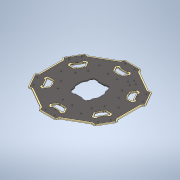
# Autodesk Inventor part: FRAME ATAS
Saved by Autodesk Inventor 2020 (Build 240168000, 168)
## iProperties
Created: 2020-03-27
Part Number: FRAME ATAS
Material: Generic
Document SubType Name: Modeling
Designer: Muhyidin
Density: 1 g/cm^3
Appearance: Carbon Fiber
Author: Muhyidin
Autodesk Inventor part; units mm, degrees
(part 1 of 2)
ref_plane "YZ Plane" through (0, 0, 0) normal (1, 0, 0) x (0, 1, 0)
ref_plane "XZ Plane" through (0, 0, 0) normal (0, 1, 0) x (-1, 0, 0)
ref_plane "XY Plane" through (0, 0, 0) normal (0, 0, 1) x (1, 0, 0)
sketch "Sketch1" plane through (0, 0, 0) normal (0, 1, 0) x (-1, 0, 0)
  circle A0 centre (15.3999, -131.0001) radius 1.6
  circle A1 centre (-15.4001, -131) radius 1.6
  line L0 (-50.3385, -87.1889) -> (-60.4808, -89.9065)
  circle A2 centre (-60.4808, -89.9065) radius 1.5
  line L1 (-50.3385, -87.1889) -> (-40.1963, -84.4713)
  line L2 (-50.3385, -87.1889) -> (-47.6209, -97.3311)
  line L3 (-50.3385, -87.1889) -> (-53.0561, -77.0467)
  circle A3 centre (-53.0561, -77.0467) radius 1.5
  circle A4 centre (-40.1963, -84.4713) radius 1.5
  circle A5 centre (-47.6209, -97.3311) radius 1.5
  line L4 (68.5102, -57.3368) -> (53.5102, -83.3176)
  line L5 (83.9102, -30.6632) -> (98.9102, -4.6824)
  line L6 (-68.5102, 57.3368) -> (-53.5102, 83.3176)
  line L7 (-83.9102, 30.6632) -> (-98.9102, 4.6824)
  line L8 (-83.9102, 30.6632) -> (-53.9102, 30.6632) construction
  circle A6 centre (98.9102, -4.6824) radius 1.6
  circle A7 centre (53.5102, -83.3176) radius 1.6
  circle A8 centre (-98.9102, 4.6824) radius 1.6
  circle A9 centre (-53.5102, 83.3176) radius 1.6
  line L9 (53.5102, -83.3176) -> (68.5102, -83.3176) construction
  circle A10 centre (0, 113) radius 1.6
  line L10 (76.2102, -44) -> (97.8609, -56.5)
  line L11 (76.2102, -44) -> (101.2102, -44) construction
  circle A11 centre (97.8609, -56.5) radius 1.6
  line L12 (-76.2102, -44) -> (-97.8609, -56.5)
  line L13 (-76.2102, -44) -> (-51.2102, -44) construction
  circle A12 centre (-97.8609, -56.5) radius 1.6
  line L14 (25, -145) -> (60, -145) construction
  line L15 (0, -138) -> (25, -138)
  line L16 (0, -138) -> (25, -138) construction
  line L17 (0, -138) -> (-25, -138)
  line L18 (0, -138) -> (25, -138) construction
  line L19 (15.4, -138) -> (22.4, -138) construction
  line L20 (-15.4, -138.0001) -> (-8.4, -138.0001) construction
  line L21 (-25, -138) -> (4.9988, -138) construction
  line L22 (-92.0115, -90.6506) -> (-87.0115, -90.6506) construction
  line L23 (-25, -138) -> (-5.0008, -138) construction
  line L24 (-25, -138) -> (-28.4202, -128.6031)
  line L25 (-25, -138) -> (-15, -138) construction
  line L26 (25, -138) -> (28.4201, -128.6031)
  line L27 (132.0114, -47.3494) -> (125.5835, -39.689)
  line L28 (107.0114, -90.6507) -> (97.1633, -88.9142)
  line L29 (111.8115, -82.3369) -> (115.3115, -76.2747) construction
  line L30 (107.0114, -90.6507) -> (117.011, -73.3308) construction
  line L31 (119.5114, -69) -> (107.0114, -90.6507)
  line L32 (107.0114, -90.6507) -> (122.0108, -64.6709) construction
  line L33 (119.5114, -69) -> (132.0114, -47.3494)
  line L34 (119.5114, -69) -> (132.0114, -47.3494) construction
  line L35 (119.5114, -69) -> (132.0114, -47.3494) construction
  circle A13 centre (121.1493, -52.1634) radius 1.6
  circle A14 centre (105.7492, -78.8369) radius 1.6
  line L36 (107.0114, 90.6505) -> (97.1634, 88.914)
  line L37 (132.0114, 47.3493) -> (125.5835, 39.6888)
  line L38 (127.2115, 55.6631) -> (123.7115, 61.7253) construction
  line L39 (132.0114, 47.3493) -> (122.0118, 64.6691) construction
  line L40 (119.5114, 68.9999) -> (132.0114, 47.3493)
  line L41 (132.0114, 47.3493) -> (117.012, 73.329) construction
  line L42 (119.5114, 68.9999) -> (107.0114, 90.6505)
  line L43 (119.5114, 68.9999) -> (107.0114, 90.6505) construction
  line L44 (119.5114, 68.9999) -> (107.0114, 90.6505) construction
  circle A15 centre (105.7494, 78.8366) radius 1.6
  circle A16 centre (121.1493, 52.163) radius 1.6
  line L45 (-25.0001, 137.9998) -> (-28.4202, 128.6029)
  line L46 (24.9999, 137.9998) -> (28.4202, 128.6029)
  line L47 (15.4, 137.9999) -> (8.4, 137.9999) construction
  line L48 (24.9999, 137.9998) -> (5.0007, 137.9998) construction
  line L49 (-0.0001, 137.9998) -> (24.9999, 137.9998)
  line L50 (24.9999, 137.9998) -> (-4.9989, 137.9998) construction
  line L51 (-0.0001, 137.9998) -> (-25.0001, 137.9998)
  line L52 (-0.0001, 137.9998) -> (-25.0001, 137.9998) construction
  line L53 (-0.0001, 137.9998) -> (-25.0001, 137.9998) construction
  circle A17 centre (-15.3999, 130.9999) radius 1.6
  circle A18 centre (15.4, 130.9999) radius 1.6
  line L54 (-132.0115, 47.3492) -> (-125.5836, 39.6889)
  line L55 (-107.0115, 90.6505) -> (-97.1634, 88.914)
  line L56 (-111.8115, 82.3367) -> (-115.3115, 76.2745) construction
  line L57 (-107.0115, 90.6505) -> (-117.0111, 73.3307) construction
  line L58 (-119.5115, 68.9999) -> (-107.0115, 90.6505)
  line L59 (-107.0115, 90.6505) -> (-122.0109, 64.6707) construction
  line L60 (-119.5115, 68.9999) -> (-132.0115, 47.3492)
  line L61 (-119.5115, 68.9999) -> (-132.0115, 47.3492) construction
  line L62 (-119.5115, 68.9999) -> (-132.0115, 47.3492) construction
  circle A19 centre (-121.1493, 52.1632) radius 1.6
  circle A20 centre (-105.7493, 78.8367) radius 1.6
  line L63 (-107.0114, -90.6507) -> (-97.1634, -88.9142)
  line L64 (-132.0114, -47.3494) -> (-125.5836, -39.689)
  line L65 (-127.2115, -55.6633) -> (-123.7115, -61.7255) construction
  line L66 (-132.0114, -47.3494) -> (-122.0118, -64.6693) construction
  line L67 (-119.5114, -69.0001) -> (-132.0114, -47.3494)
  line L68 (-132.0114, -47.3494) -> (-117.012, -73.3292) construction
  line L69 (-119.5114, -69.0001) -> (-107.0114, -90.6507)
  line L70 (-119.5114, -69.0001) -> (-107.0114, -90.6507) construction
  line L71 (-119.5114, -69.0001) -> (-107.0114, -90.6507) construction
  circle A21 centre (-105.7494, -78.8368) radius 1.6
  circle A22 centre (-121.1493, -52.1632) radius 1.6
  line L72 (-28.4202, -128.6031) -> (-97.1634, -88.9142)
  line L73 (97.1633, -88.9142) -> (28.4201, -128.6031)
  line L74 (125.5835, 39.6888) -> (125.5835, -39.689)
  line L75 (28.4202, 128.6029) -> (97.1634, 88.914)
  line L76 (-97.1634, 88.914) -> (-28.4202, 128.6029)
  line L77 (-125.5836, -39.689) -> (-125.5836, 39.6889)
  line L78 (-15.4, -131) -> (42.1, -131) construction
  circle A23 centre (15.4, -73.5001) radius 1.65
  circle A24 centre (-15.4001, -73.5) radius 1.65
  circle A25 centre (71.3528, -23.4133) radius 1.65
  circle A26 centre (55.9528, -50.0869) radius 1.65
  circle A27 centre (55.9528, 50.0867) radius 1.65
  circle A28 centre (71.3528, 23.413) radius 1.65
  circle A29 centre (-15.4, 73.4999) radius 1.65
  circle A30 centre (15.4, 73.4999) radius 1.65
  circle A31 centre (-71.3529, 23.4131) radius 1.65
  circle A32 centre (-55.9528, 50.0867) radius 1.65
  circle A33 centre (-55.9529, -50.0869) radius 1.65
  circle A34 centre (-71.3529, -23.4132) radius 1.65
  line L79 (36.5897, -0.0001) -> (36.5897, -10.9001)
  line L80 (36.5897, -0.0001) -> (47.4897, -0.0001) construction
  line L81 (36.5897, -10.9001) -> (30.2097, -21.9505)
  line L82 (36.5897, -10.9001) -> (49.3497, -10.9001) construction
  line L83 (30.2097, -21.9505) -> (30.2097, -30.6505)
  line L84 (30.2097, -21.9505) -> (38.9097, -21.9505) construction
  line L85 (30.2097, -30.6505) -> (23.4386, -38.72)
  line L86 (30.2097, -30.6505) -> (40.7437, -30.6505) construction
  line L87 (23.4386, -38.72) -> (12.9386, -38.72)
  line L88 (12.9386, -38.72) -> (11.0102, -36.4219)
  line L89 (0, -88.9499) -> (6, -88.9499)
  line L90 (6, -88.9499) -> (8.5, -88.9499) construction
  line L91 (6, -88.9499) -> (7.9151, -90.5569)
  line L92 (6, -88.9499) -> (8.5, -88.9499) construction
  line L93 (7.9151, -90.5569) -> (14.9151, -90.5569)
  line L94 (14.9151, -90.5569) -> (24.9151, -107.8774)
  line L95 (14.9151, -90.5569) -> (34.9151, -90.5569) construction
  line L96 (24.9151, -107.8774) -> (19.1301, -114.7719)
  line L97 (24.9151, -115.3493) -> (33.9151, -115.3493) construction
  line L98 (19.1301, -114.7719) -> (13.35, -114.7719)
  line L99 (19.1301, -114.7719) -> (24.9101, -114.7719) construction
  line L100 (13.35, -114.7719) -> (11.1, -110.8748)
  line L101 (13.35, -114.7719) -> (17.85, -114.7719) construction
  line L102 (11.1, -110.8748) -> (0, -110.8748)
  line L103 (0, -88.9499) -> (-6, -88.95)
  line L104 (-6, -88.95) -> (-8.5, -88.95) construction
  line L105 (-6, -88.95) -> (-7.9151, -90.557)
  line L106 (-6, -88.95) -> (-8.5, -88.95) construction
  line L107 (-7.9151, -90.557) -> (-14.9151, -90.557)
  line L108 (-14.9151, -90.557) -> (-24.9151, -107.8775)
  line L109 (-14.9151, -90.557) -> (-34.9151, -90.557) construction
  line L110 (-24.9151, -107.8775) -> (-19.13, -114.7719)
  line L111 (-19.13, -114.7719) -> (-13.35, -114.7719)
  line L112 (-19.13, -114.7719) -> (-24.91, -114.7719) construction
  line L113 (-13.35, -114.7719) -> (-11.1, -110.8748)
  line L114 (-13.35, -114.7719) -> (-17.85, -114.7719) construction
  line L115 (-11.1, -110.8748) -> (0, -110.8748)
  line L116 (101.5703, -45.8245) -> (96.0203, -55.4374)
  line L117 (90.4703, -65.0503) -> (96.0203, -55.4374)
  line L118 (92.7203, -68.9474) -> (90.4703, -65.0503)
  line L119 (92.7203, -68.9474) -> (90.4703, -72.8445) construction
  line L120 (70.967, -58.1954) -> (60.967, -75.5159) construction
  line L121 (89.8303, -73.953) -> (86.9403, -78.9587) construction
  line L122 (80.967, -75.5159) -> (89.8303, -73.953)
  line L123 (89.8303, -73.953) -> (92.7203, -68.9474)
  line L124 (70.967, -58.1954) -> (80.967, -75.5159)
  line L125 (77.0328, -44.475) -> (74.0329, -49.6712)
  line L126 (74.0329, -49.6712) -> (72.7829, -51.8362) construction
  line L127 (74.0329, -49.6712) -> (72.7829, -51.8362) construction
  line L128 (74.0329, -49.6712) -> (74.467, -52.1332)
  line L129 (74.467, -52.1332) -> (70.967, -58.1954)
  line L130 (108.9603, -40.8188) -> (111.8503, -35.8132) construction
  line L131 (105.882, -32.3616) -> (108.9603, -40.8188)
  line L132 (85.882, -32.3616) -> (95.882, -15.0411) construction
  line L133 (85.882, -32.3616) -> (105.882, -32.3616)
  line L134 (108.9603, -40.8188) -> (106.0703, -45.8245)
  line L135 (106.0703, -45.8245) -> (108.3203, -41.9274) construction
  line L136 (106.0703, -45.8245) -> (101.5703, -45.8245)
  line L137 (80.0328, -39.2789) -> (81.2828, -37.1138) construction
  line L138 (80.0328, -39.2789) -> (82.382, -38.4238)
  line L139 (80.0328, -39.2789) -> (81.2828, -37.1138) construction
  line L140 (77.0328, -44.475) -> (80.0328, -39.2789)
  line L141 (82.382, -38.4238) -> (85.882, -32.3616)
  line L142 (90.4702, 65.0502) -> (96.0202, 55.4373)
  line L143 (101.5702, 45.8244) -> (96.0202, 55.4373)
  line L144 (106.0702, 45.8244) -> (101.5702, 45.8244)
  line L145 (106.0702, 45.8244) -> (108.3202, 41.9273) construction
  line L146 (85.8821, 32.3615) -> (95.8821, 15.041) construction
  line L147 (108.9603, 40.8188) -> (111.8503, 35.8131) construction
  line L148 (105.8821, 32.3615) -> (108.9603, 40.8188)
  line L149 (108.9603, 40.8188) -> (106.0702, 45.8244)
  line L150 (85.8821, 32.3615) -> (105.8821, 32.3615)
  line L151 (77.0328, 44.4748) -> (80.0328, 39.2788)
  line L152 (80.0328, 39.2788) -> (81.2828, 37.1137) construction
  line L153 (80.0328, 39.2788) -> (81.2828, 37.1137) construction
  line L154 (80.0328, 39.2788) -> (82.3821, 38.4237)
  line L155 (82.3821, 38.4237) -> (85.8821, 32.3615)
  line L156 (89.8302, 73.953) -> (86.9402, 78.9586) construction
  line L157 (80.9669, 75.5157) -> (89.8302, 73.953)
  line L158 (70.9669, 58.1952) -> (60.9669, 75.5157) construction
  line L159 (70.9669, 58.1952) -> (80.9669, 75.5157)
  line L160 (89.8302, 73.953) -> (92.7202, 68.9473)
  line L161 (92.7202, 68.9473) -> (90.4702, 72.8444) construction
  line L162 (92.7202, 68.9473) -> (90.4702, 65.0502)
  line L163 (74.0328, 49.671) -> (72.7828, 51.8361) construction
  line L164 (74.0328, 49.671) -> (74.4669, 52.133)
  line L165 (74.0328, 49.671) -> (72.7828, 51.8361) construction
  line L166 (77.0328, 44.4748) -> (74.0328, 49.671)
  line L167 (74.4669, 52.133) -> (70.9669, 58.1952)
  line L168 (-11.1001, 110.8746) -> (-0.0001, 110.8746)
  line L169 (11.0999, 110.8746) -> (-0.0001, 110.8746)
  line L170 (13.3499, 114.7717) -> (11.0999, 110.8746)
  line L171 (13.3499, 114.7717) -> (17.8499, 114.7717) construction
  line L172 (14.915, 90.5568) -> (34.915, 90.5568) construction
  line L173 (19.13, 114.7717) -> (24.91, 114.7717) construction
  line L174 (24.915, 107.8773) -> (19.13, 114.7717)
  line L175 (19.13, 114.7717) -> (13.3499, 114.7717)
  line L176 (14.915, 90.5568) -> (24.915, 107.8773)
  line L177 (0, 88.9498) -> (5.9999, 88.9498)
  line L178 (5.9999, 88.9498) -> (8.4999, 88.9498) construction
  line L179 (5.9999, 88.9498) -> (8.4999, 88.9498) construction
  line L180 (5.9999, 88.9498) -> (7.915, 90.5568)
  line L181 (7.915, 90.5568) -> (14.915, 90.5568)
  line L182 (-19.1301, 114.7717) -> (-24.9102, 114.7717) construction
  line L183 (-24.9151, 107.8773) -> (-19.1301, 114.7717)
  line L184 (-14.9151, 90.5567) -> (-34.9151, 90.5567) construction
  line L185 (-14.9151, 90.5567) -> (-24.9151, 107.8773)
  line L186 (-19.1301, 114.7717) -> (-13.3501, 114.7717)
  line L187 (-13.3501, 114.7717) -> (-17.8501, 114.7717) construction
  line L188 (-13.3501, 114.7717) -> (-11.1001, 110.8746)
  line L189 (-6, 88.9498) -> (-8.5001, 88.9498) construction
  line L190 (-6, 88.9498) -> (-7.9151, 90.5567)
  line L191 (-6, 88.9498) -> (-8.5, 88.9498) construction
  line L192 (0, 88.9498) -> (-6, 88.9498)
  line L193 (-7.9151, 90.5567) -> (-14.9151, 90.5567)
  line L194 (-101.5703, 45.8243) -> (-96.0203, 55.4372)
  line L195 (-90.4703, 65.0501) -> (-96.0203, 55.4372)
  line L196 (-92.7203, 68.9472) -> (-90.4703, 65.0501)
  line L197 (-92.7203, 68.9472) -> (-90.4703, 72.8443) construction
  line L198 (-70.9671, 58.1952) -> (-60.9671, 75.5157) construction
  line L199 (-89.8303, 73.9529) -> (-86.9403, 78.9585) construction
  line L200 (-80.9671, 75.5157) -> (-89.8303, 73.9529)
  line L201 (-89.8303, 73.9529) -> (-92.7203, 68.9472)
  line L202 (-70.9671, 58.1952) -> (-80.9671, 75.5157)
  line L203 (-77.0329, 44.4748) -> (-74.0329, 49.671)
  line L204 (-74.0329, 49.671) -> (-72.7829, 51.8361) construction
  line L205 (-74.0329, 49.671) -> (-72.7829, 51.8361) construction
  line L206 (-74.0329, 49.671) -> (-74.4671, 52.133)
  line L207 (-74.4671, 52.133) -> (-70.9671, 58.1952)
  line L208 (-108.9604, 40.8187) -> (-111.8504, 35.813) construction
  line L209 (-105.8821, 32.3615) -> (-108.9604, 40.8187)
  line L210 (-85.8821, 32.3615) -> (-95.8821, 15.041) construction
  line L211 (-85.8821, 32.3615) -> (-105.8821, 32.3615)
  line L212 (-108.9604, 40.8187) -> (-106.0703, 45.8243)
  line L213 (-106.0703, 45.8243) -> (-108.3203, 41.9272) construction
  line L214 (-106.0703, 45.8243) -> (-101.5703, 45.8243)
  line L215 (-80.0329, 39.2787) -> (-81.2829, 37.1136) construction
  line L216 (-80.0329, 39.2787) -> (-82.3821, 38.4236)
  line L217 (-80.0329, 39.2787) -> (-81.2829, 37.1136) construction
  line L218 (-77.0329, 44.4748) -> (-80.0329, 39.2787)
  line L219 (-82.3821, 38.4236) -> (-85.8821, 32.3615)
  line L220 (-90.4703, -65.0503) -> (-96.0203, -55.4375)
  line L221 (-101.5703, -45.8246) -> (-96.0203, -55.4375)
  line L222 (-106.0703, -45.8246) -> (-101.5703, -45.8246)
  line L223 (-106.0703, -45.8246) -> (-108.3203, -41.9275) construction
  line L224 (-85.8821, -32.3617) -> (-95.8821, -15.0412) construction
  line L225 (-108.9603, -40.8189) -> (-111.8503, -35.8133) construction
  line L226 (-105.8821, -32.3617) -> (-108.9603, -40.8189)
  line L227 (-108.9603, -40.8189) -> (-106.0703, -45.8246)
  line L228 (-85.8821, -32.3617) -> (-105.8821, -32.3617)
  line L229 (-77.0329, -44.475) -> (-80.0329, -39.2789)
  line L230 (-80.0329, -39.2789) -> (-81.2829, -37.1139) construction
  line L231 (-80.0329, -39.2789) -> (-81.2829, -37.1139) construction
  line L232 (-80.0329, -39.2789) -> (-82.3821, -38.4239)
  line L233 (-82.3821, -38.4239) -> (-85.8821, -32.3617)
  line L234 (-89.8303, -73.9531) -> (-86.9402, -78.9588) construction
  line L235 (-80.967, -75.5159) -> (-89.8303, -73.9531)
  line L236 (-70.967, -58.1954) -> (-60.967, -75.5159) construction
  line L237 (-70.967, -58.1954) -> (-80.967, -75.5159)
  line L238 (-89.8303, -73.9531) -> (-92.7203, -68.9475)
  line L239 (-92.7203, -68.9475) -> (-90.4703, -72.8446) construction
  line L240 (-92.7203, -68.9475) -> (-90.4703, -65.0503)
  line L241 (-74.0329, -49.6712) -> (-72.7829, -51.8363) construction
  line L242 (-74.0329, -49.6712) -> (-74.467, -52.1332)
  line L243 (-74.0329, -49.6712) -> (-72.7829, -51.8362) construction
  line L244 (-77.0329, -44.475) -> (-74.0329, -49.6712)
  line L245 (-74.467, -52.1332) -> (-70.967, -58.1954)
  line L246 (0, -88.9499) -> (0, -36.4219)
  line L247 (0, -91.9499) -> (5.9999, -91.9499)
  line L248 (5.9999, -91.9499) -> (7.532, -93.2355)
  line L249 (5.9999, -91.9499) -> (7.9999, -91.9499) construction
  line L250 (7.532, -93.2355) -> (12.532, -93.2355)
  line L251 (12.532, -93.2355) -> (20.032, -106.2259)
  line L252 (20.032, -106.2259) -> (16.8181, -110.0561)
  line L253 (16.8181, -110.0561) -> (13.8181, -110.0561)
  line L254 (13.8181, -110.0561) -> (12.5681, -107.8911)
  line L255 (12.5681, -107.8911) -> (0, -107.8911)
  line L256 (0, -91.9499) -> (-6, -91.9499)
  line L257 (-6, -91.9499) -> (-7.5321, -93.2355)
  line L258 (-6, -91.9499) -> (-8, -91.9499) construction
  line L259 (-7.5321, -93.2355) -> (-12.5321, -93.2355)
  line L260 (-12.5321, -93.2355) -> (-20.0321, -106.2259)
  line L261 (-20.0321, -106.2259) -> (-16.8181, -110.0561)
  line L262 (-16.8181, -110.0561) -> (-13.8181, -110.0561)
  line L263 (-13.8181, -110.0561) -> (-12.5681, -107.8911)
  line L264 (-12.5681, -107.8911) -> (0, -107.8911)
  line L265 (79.6309, -45.975) -> (76.6309, -51.1711)
  line L266 (76.9782, -53.1407) -> (74.4782, -57.4709)
  line L267 (76.6309, -51.1711) -> (76.9782, -53.1407)
  line L268 (88.4022, -66.9949) -> (87.1522, -64.8299)
  line L269 (87.1522, -64.8299) -> (93.4363, -53.9456)
  line L270 (81.9782, -70.4613) -> (86.9022, -69.593)
  line L271 (86.9022, -69.593) -> (88.4022, -66.9949)
  line L272 (74.4782, -57.4709) -> (81.9782, -70.4613)
  line L273 (82.6309, -40.7789) -> (83.6309, -39.0468) construction
  line L274 (82.6309, -40.7789) -> (84.5103, -40.0949)
  line L275 (79.6309, -45.975) -> (82.6309, -40.7789)
  line L276 (84.5103, -40.0949) -> (87.0103, -35.7647)
  line L277 (87.0103, -35.7647) -> (102.0103, -35.7647)
  line L278 (103.7204, -40.4632) -> (102.2204, -43.0613)
  line L279 (102.2204, -43.0613) -> (99.7204, -43.0613)
  line L280 (102.0103, -35.7647) -> (103.7204, -40.4632)
  line L281 (99.7204, -43.0613) -> (93.4363, -53.9456)
  line L282 (79.6309, 45.9748) -> (82.6309, 40.7787)
  line L283 (84.5103, 40.0947) -> (87.0103, 35.7646)
  line L284 (82.6309, 40.7787) -> (84.5103, 40.0947)
  line L285 (102.2204, 43.0611) -> (99.7204, 43.0611)
  line L286 (99.7204, 43.0611) -> (93.4363, 53.9454)
  line L287 (102.0103, 35.7646) -> (103.7204, 40.463)
  line L288 (103.7204, 40.463) -> (102.2204, 43.0611)
  line L289 (87.0103, 35.7646) -> (102.0103, 35.7646)
  line L290 (76.6309, 51.171) -> (75.6309, 52.903) construction
  line L291 (76.6309, 51.171) -> (76.9782, 53.1406)
  line L292 (79.6309, 45.9748) -> (76.6309, 51.171)
  line L293 (76.9782, 53.1406) -> (74.4782, 57.4707)
  line L294 (74.4782, 57.4707) -> (81.9782, 70.4611)
  line L295 (86.9022, 69.5928) -> (88.4022, 66.9948)
  line L296 (88.4022, 66.9948) -> (87.1522, 64.8297)
  line L297 (81.9782, 70.4611) -> (86.9022, 69.5928)
  line L298 (87.1522, 64.8297) -> (93.4363, 53.9454)
  line L299 (0, 91.9498) -> (5.9999, 91.9498)
  line L300 (7.532, 93.2354) -> (12.532, 93.2354)
  line L301 (5.9999, 91.9498) -> (7.532, 93.2354)
  line L302 (13.8181, 110.056) -> (12.5681, 107.8909)
  line L303 (12.5681, 107.8909) -> (0, 107.8909)
  line L304 (20.032, 106.2257) -> (16.8181, 110.056)
  line L305 (16.8181, 110.056) -> (13.8181, 110.056)
  line L306 (12.532, 93.2354) -> (20.032, 106.2257)
  line L307 (-6, 91.9498) -> (-8, 91.9498) construction
  line L308 (-6, 91.9498) -> (-7.5321, 93.2354)
  line L309 (0, 91.9498) -> (-6, 91.9498)
  line L310 (-7.5321, 93.2354) -> (-12.5321, 93.2354)
  line L311 (-12.5321, 93.2354) -> (-20.0321, 106.2257)
  line L312 (-16.8181, 110.056) -> (-13.8181, 110.056)
  line L313 (-13.8181, 110.056) -> (-12.5681, 107.8909)
  line L314 (-20.0321, 106.2257) -> (-16.8181, 110.056)
  line L315 (-12.5681, 107.8909) -> (0, 107.8909)
  line L316 (-79.6309, 45.9748) -> (-76.631, 51.171)
  line L317 (-76.9783, 53.1406) -> (-74.4783, 57.4707)
  line L318 (-76.631, 51.171) -> (-76.9783, 53.1406)
  line L319 (-88.4023, 66.9948) -> (-87.1523, 64.8297)
  line L320 (-87.1523, 64.8297) -> (-93.4364, 53.9454)
  line L321 (-81.9783, 70.4611) -> (-86.9023, 69.5928)
  line L322 (-86.9023, 69.5928) -> (-88.4023, 66.9948)
  line L323 (-74.4783, 57.4707) -> (-81.9783, 70.4611)
  line L324 (-82.6309, 40.7787) -> (-83.6309, 39.0467) construction
  line L325 (-82.6309, 40.7787) -> (-84.5103, 40.0947)
  line L326 (-79.6309, 45.9748) -> (-82.6309, 40.7787)
  line L327 (-84.5103, 40.0947) -> (-87.0103, 35.7646)
  line L328 (-87.0103, 35.7646) -> (-102.0103, 35.7646)
  line L329 (-103.7204, 40.463) -> (-102.2204, 43.0611)
  line L330 (-102.2204, 43.0611) -> (-99.7204, 43.0611)
  line L331 (-102.0103, 35.7646) -> (-103.7204, 40.463)
  line L332 (-99.7204, 43.0611) -> (-93.4364, 53.9454)
  line L333 (-79.6309, -45.975) -> (-82.6309, -40.7789)
  line L334 (-84.5103, -40.0949) -> (-87.0103, -35.7647)
  line L335 (-82.6309, -40.7789) -> (-84.5103, -40.0949)
  line L336 (-102.2204, -43.0613) -> (-99.7204, -43.0613)
  line L337 (-99.7204, -43.0613) -> (-93.4364, -53.9456)
  line L338 (-102.0103, -35.7647) -> (-103.7204, -40.4632)
  line L339 (-103.7204, -40.4632) -> (-102.2204, -43.0613)
  line L340 (-87.0103, -35.7647) -> (-102.0103, -35.7647)
  line L341 (-76.631, -51.1711) -> (-75.631, -52.9032) construction
  line L342 (-76.631, -51.1711) -> (-76.9783, -53.1407)
  line L343 (-79.6309, -45.975) -> (-76.631, -51.1711)
  line L344 (-76.9783, -53.1407) -> (-74.4783, -57.4709)
  line L345 (-74.4783, -57.4709) -> (-81.9783, -70.4613)
  line L346 (-86.9023, -69.593) -> (-88.4023, -66.9949)
  line L347 (-88.4023, -66.9949) -> (-87.1523, -64.8299)
  line L348 (-81.9783, -70.4613) -> (-86.9023, -69.593)
  line L349 (-87.1523, -64.8299) -> (-93.4364, -53.9456)
  line L350 (0, -138) -> (0, -141)
  line L351 (0, -138) -> (3, -138) construction
  line L352 (-25, -138) -> (-22, -138) construction
  line L353 (-25, -138) -> (-20, -138) construction
  line L354 (0, -141) -> (-27.5173, -141)
  line L355 (0, -141) -> (27.5173, -141) construction
  line L356 (-27.5173, -141) -> (-13.8071, -141) construction
  line L357 (-28.4202, -128.6031) -> (-34.2721, -128.6031)
  line L358 (-28.4202, -128.6031) -> (-22.5683, -128.6031) construction
  line L359 (-107.0114, -90.6507) -> (-104.0114, -90.6507) construction
  line L360 (-27.5173, -141) -> (-30.9375, -131.6031)
  line L361 (-27.5173, -141) -> (-17.5173, -141) construction
  line L362 (0, -141) -> (27.5173, -141)
  line L363 (27.5173, -141) -> (13.8071, -141) construction
  line L364 (27.5173, -141) -> (30.9375, -131.6031)
  line L365 (108.3508, -94.3307) -> (98.5028, -92.5942)
  line L366 (122.1095, -70.5) -> (108.3508, -94.3307)
  line L367 (122.1095, -70.5) -> (135.8681, -46.6693) construction
  line L368 (122.1095, -70.5) -> (135.8681, -46.6693)
  line L369 (135.8681, -46.6693) -> (129.4403, -39.0089)
  line L370 (135.8681, 46.6692) -> (129.4402, 39.0088)
  line L371 (122.1095, 70.4999) -> (135.8681, 46.6692)
  line L372 (122.1095, 70.4999) -> (108.3508, 94.3306) construction
  line L373 (122.1095, 70.4999) -> (108.3508, 94.3306)
  line L374 (108.3508, 94.3306) -> (98.5027, 92.5941)
  line L375 (27.5172, 140.9998) -> (30.9374, 131.6029)
  line L376 (-0.0001, 140.9998) -> (27.5172, 140.9998)
  line L377 (-0.0001, 140.9998) -> (-27.5173, 140.9998) construction
  line L378 (-0.0001, 140.9998) -> (-27.5173, 140.9998)
  line L379 (-27.5173, 140.9998) -> (-30.9376, 131.6029)
  line L380 (-108.3509, 94.3305) -> (-98.5028, 92.5941)
  line L381 (-122.1095, 70.4999) -> (-108.3509, 94.3305)
  line L382 (-122.1095, 70.4999) -> (-135.8682, 46.6692) construction
  line L383 (-122.1095, 70.4999) -> (-135.8682, 46.6692)
  line L384 (-135.8682, 46.6692) -> (-129.4403, 39.0087)
  line L385 (-135.8682, -46.6694) -> (-129.4403, -39.0089)
  line L386 (-122.1095, -70.5001) -> (-135.8682, -46.6694)
  line L387 (-122.1095, -70.5001) -> (-108.3509, -94.3307) construction
  line L388 (-122.1095, -70.5001) -> (-108.3509, -94.3307)
  line L389 (-108.3509, -94.3307) -> (-98.5028, -92.5943)
  line L390 (-30.9375, -131.6031) -> (-98.5028, -92.5943)
  line L391 (98.5028, -92.5942) -> (30.9375, -131.6031)
  line L392 (129.4402, 39.0088) -> (129.4403, -39.0089)
  line L393 (30.9374, 131.6029) -> (98.5027, 92.5941)
  line L394 (-98.5028, 92.5941) -> (-30.9376, 131.6029)
  line L395 (-129.4403, -39.0089) -> (-129.4403, 39.0087)
  line L396 (11.0102, -36.4219) -> (0, -36.4219)
  line L397 (-36.5897, -0.0001) -> (-36.5897, -10.9001)
  line L398 (-36.5897, -10.9001) -> (-30.2097, -21.9505)
  line L399 (-36.5897, -10.9001) -> (-49.3497, -10.9001) construction
  line L400 (-30.2097, -21.9505) -> (-30.2097, -30.6505)
  line L401 (-30.2097, -21.9505) -> (-38.9097, -21.9505) construction
  line L402 (-30.2097, -30.6505) -> (-23.4386, -38.72)
  line L403 (-23.4386, -38.72) -> (-12.9386, -38.72)
  line L404 (-12.9386, -38.72) -> (-11.0102, -36.4219)
  line L405 (-11.0102, -36.4219) -> (0, -36.4219)
  line L406 (36.5897, -0.0001) -> (36.5897, 10.8999)
  line L407 (36.5897, 10.8999) -> (30.2097, 21.9504)
  line L408 (36.5897, 10.8999) -> (49.3497, 10.8999) construction
  line L409 (30.2097, 21.9504) -> (30.2097, 30.6504)
  line L410 (30.2097, 21.9504) -> (38.9097, 21.9504) construction
  line L411 (30.2097, 30.6504) -> (23.4386, 38.7199)
  line L412 (23.4386, 38.7199) -> (12.9386, 38.7199)
  line L413 (12.9386, 38.7199) -> (11.0102, 36.4218)
  line L414 (11.0102, 36.4218) -> (0, 36.4218)
  line L415 (-23.4386, 38.7199) -> (-12.9386, 38.7199)
  line L416 (-30.2097, 30.6504) -> (-23.4386, 38.7199)
  line L417 (-11.0102, 36.4218) -> (0, 36.4218)
  line L418 (-12.9386, 38.7199) -> (-11.0102, 36.4218)
  line L419 (-30.2097, 21.9504) -> (-30.2097, 30.6504)
  line L420 (-30.2097, 21.9504) -> (-38.9097, 21.9504) construction
  line L421 (-36.5897, 10.8999) -> (-30.2097, 21.9504)
  line L422 (-36.5897, 10.8999) -> (-49.3497, 10.8999) construction
  line L423 (-36.5897, -0.0001) -> (-36.5897, 10.8999)
  point P0 (0, -0.0001)
  point P1 (-50.3385, -87.1889)
  point P2 (-50.3385, -87.1889)
  point P3 (-50.3385, -87.1889)
  point P4 (-50.3385, -87.1889)
  point P5 (-50.3385, -87.1889)
  point P6 (28.4201, -128.6031)
  point P7 (-28.4202, 128.6029)
  dimension "d427" = 3.2
  dimension "d428" = 3.2
  dimension "d473" = 10.5
  dimension "d474" = 3
  dimension "d479" = 10.5
  dimension "d480" = 10.5
  dimension "d481" = 10.5
  dimension "d486" = 3
  dimension "d491" = 3
  dimension "d496" = 3
  dimension "d497" = 30
  dimension "d498" = 30
  dimension "d499" = 30
  dimension "d500" = 30
  dimension "d501" = 120
  dimension "d597" = 25
  dimension "d598" = 30
  dimension "d603" = 25
  dimension "d604" = 150
  dimension "d625" = 0
  dimension "d627" = 180
  dimension "d646" = 10
  dimension "d647" = 110
  dimension "d650" = 360
  dimension "d655" = 360
  dimension "d659" = 3.3
  dimension "d664" = 3.3
  dimension "d667" = 360
  dimension "d672" = 10.9
  dimension "d673" = 90
  dimension "d674" = 12.76
  dimension "d675" = 120
  dimension "d676" = 8.7
  dimension "d677" = 90
  dimension "d678" = 10.534
  dimension "d679" = 130
  dimension "d680" = 10.5
  dimension "d681" = 3
  dimension "d684" = 6
  dimension "d687" = 2.5
  dimension "d688" = 40
  dimension "d689" = 7
  dimension "d690" = 20
  dimension "d691" = 60
  dimension "d692" = 9
  dimension "d693" = 129.999
  dimension "d695" = 180
  dimension "d696" = 4.5
  dimension "d697" = 120
  dimension "d701" = 360
  dimension "d705" = 3
  dimension "d706" = 2
  dimension "d707" = 40
  dimension "d708" = 5
  dimension "d709" = 140
  dimension "d710" = 15
  dimension "d711" = 120
  dimension "d712" = 5
  dimension "d713" = 110
  dimension "d714" = 3
  dimension "d715" = 130
  dimension "d716" = 2.5
  dimension "d717" = 120
  dimension "d720" = 360
  constraints: 848 end point, 41 horizontal, 35 centre point, 20 equal length, 10 symmetric about line, 3 parallel, 3 vertical, 2 coincident, 2 perpendicular, 787 other
  measures "d427" diameter of A0
  measures "d428" diameter of A1
  measures "d473" distance of L0.end L0.start
  measures "d474" diameter of A2
  measures "d479" distance of L1.start L1.end
  measures "d480" distance of L1.start L2.end
  measures "d481" distance of L1.start L3.end
  measures "d486" diameter of A3
  measures "d491" diameter of A4
  measures "d496" diameter of A5
  measures "d497" distance of L4.start L4.end
  measures "d498" distance of L5.start L5.end
  measures "d499" distance of L6.start L6.end
  measures "d500" distance of L7.start L7.end
  measures "d501" angle of L7 L8
  measures "d597" distance of L10.start L10.end
  measures "d598" angle of L10 L11
  measures "d603" distance of L12.start L12.end
  measures "d604" angle of L12 L13
  measures "d625" distance between parallel lines of L15 L16
  measures "d627" angle of L17 L18
  measures "d646" distance of L17.end L24.end
  measures "d647" angle of L25 L24
  measures "d659" diameter of A23
  measures "d664" diameter of A24
  measures "d672" distance of L79.start L79.end
  measures "d673" angle of L79 L80
  measures "d674" distance of L79.end L81.end
  measures "d675" angle of L81 L82
  measures "d676" distance of L81.end L83.end
  measures "d677" angle of L83 L84
  measures "d678" distance of L83.end L85.end
  measures "d679" angle of L85 L86
  measures "d680" distance of L85.end L87.end
  measures "d681" distance of L87.end L88.end
  measures "d684" distance of L89.start L89.end
  measures "d687" distance of L89.end L91.end
  measures "d688" angle of L91 L92
  measures "d689" distance of L91.end L93.end
  measures "d690" distance of L93.end L94.end
  measures "d691" angle of L94 L95
  measures "d692" distance of L94.end L96.end
  measures "d693" angle of L96 L97
  measures "d695" angle of L98 L99
  measures "d696" distance of L98.end L100.end
  measures "d697" angle of L101 L100
  measures "d705" distance of L89.start L247.start
  measures "d706" distance of L247.end L248.end
  measures "d707" angle of L248 L249
  measures "d708" distance of L248.end L250.end
  measures "d709" angle of L250 L248
  measures "d710" distance of L250.end L251.end
  measures "d711" angle of L250 L251
  measures "d712" distance of L251.end L252.end
  measures "d713" angle of L251 L252
  measures "d714" distance of L252.end L253.end
  measures "d715" angle of L252 L253
  measures "d716" distance of L253.end L254.end
  measures "d717" angle of L253 L254
extrude "Extrusion11" add sketch "Sketch1" along normal blind 3 contours L17 L24 L72 L63 L69 L67 L64 L77 L54 L60 L58 L55 L76 L45 L51 L49 L46 L75 L36 L42 L40 L37 L74 L27 L33 L31 L28 L73 L26 L15
sketch "Sketch3" plane through (0, 3, 0) normal (0, 1, 0) x (1, 0, 0)
  circle A0 centre (15.3999, -131.0001) radius 1.6
  circle A1 centre (-15.4001, -131) radius 1.6
  circle A2 centre (-60.4808, -89.9065) radius 1.5
  line L0 (-50.3385, -87.1889) -> (-60.4808, -89.9065)
  line L1 (-50.3385, -87.1889) -> (-40.1963, -84.4713)
  line L2 (-50.3385, -87.1889) -> (-47.6209, -97.3311)
  line L3 (-50.3385, -87.1889) -> (-53.0561, -77.0467)
  circle A3 centre (-53.0561, -77.0467) radius 1.5
  circle A4 centre (-40.1963, -84.4713) radius 1.5
  circle A5 centre (-47.6209, -97.3311) radius 1.5
  line L4 (68.5102, -57.3368) -> (53.5102, -83.3176)
  line L5 (83.9102, -30.6632) -> (98.9102, -4.6824)
  line L6 (-68.5102, 57.3368) -> (-53.5102, 83.3176)
  line L7 (-83.9102, 30.6632) -> (-98.9102, 4.6824)
  line L8 (-83.9102, 30.6632) -> (-53.9102, 30.6632) construction
  circle A6 centre (98.9102, -4.6824) radius 1.6
  circle A7 centre (53.5102, -83.3176) radius 1.6
  circle A8 centre (-98.9102, 4.6824) radius 1.6
  circle A9 centre (-53.5102, 83.3176) radius 1.6
  line L9 (53.5102, -83.3176) -> (68.5102, -83.3176) construction
  circle A10 centre (0, 113) radius 1.6
  line L10 (76.2102, -44) -> (97.8609, -56.5)
  line L11 (76.2102, -44) -> (101.2102, -44) construction
  circle A11 centre (97.8609, -56.5) radius 1.6
  line L12 (-76.2102, -44) -> (-97.8609, -56.5)
  line L13 (-76.2102, -44) -> (-51.2102, -44) construction
  circle A12 centre (-97.8609, -56.5) radius 1.6
  line L14 (25, -145) -> (60, -145) construction
  line L15 (0, -138) -> (25, -138)
  line L16 (0, -138) -> (25, -138) construction
  line L17 (0, -138) -> (-25, -138)
  line L18 (0, -138) -> (25, -138) construction
  line L19 (15.4, -138) -> (22.4, -138) construction
  line L20 (-15.4, -138.0001) -> (-8.4, -138.0001) construction
  line L21 (-25, -138) -> (4.9988, -138) construction
  line L22 (-92.0115, -90.6506) -> (-87.0115, -90.6506) construction
  line L23 (-25, -138) -> (-5.0008, -138) construction
  line L24 (-25, -138) -> (-28.4202, -128.6031)
  line L25 (-25, -138) -> (-15, -138) construction
  line L26 (25, -138) -> (28.4201, -128.6031)
  line L27 (132.0114, -47.3494) -> (125.5835, -39.689)
  line L28 (107.0114, -90.6507) -> (97.1633, -88.9142)
  line L29 (111.8115, -82.3369) -> (115.3115, -76.2747) construction
  line L30 (107.0114, -90.6507) -> (117.011, -73.3308) construction
  line L31 (119.5114, -69) -> (107.0114, -90.6507)
  line L32 (107.0114, -90.6507) -> (122.0108, -64.6709) construction
  line L33 (119.5114, -69) -> (132.0114, -47.3494)
  line L34 (119.5114, -69) -> (132.0114, -47.3494) construction
  line L35 (119.5114, -69) -> (132.0114, -47.3494) construction
  circle A13 centre (121.1493, -52.1634) radius 1.6
  circle A14 centre (105.7492, -78.8369) radius 1.6
  line L36 (107.0114, 90.6505) -> (97.1634, 88.914)
  line L37 (132.0114, 47.3493) -> (125.5835, 39.6888)
  line L38 (127.2115, 55.6631) -> (123.7115, 61.7253) construction
  line L39 (132.0114, 47.3493) -> (122.0118, 64.6691) construction
  line L40 (119.5114, 68.9999) -> (132.0114, 47.3493)
  line L41 (132.0114, 47.3493) -> (117.012, 73.329) construction
  line L42 (119.5114, 68.9999) -> (107.0114, 90.6505)
  line L43 (119.5114, 68.9999) -> (107.0114, 90.6505) construction
  line L44 (119.5114, 68.9999) -> (107.0114, 90.6505) construction
  circle A15 centre (105.7494, 78.8366) radius 1.6
  circle A16 centre (121.1493, 52.163) radius 1.6
  line L45 (-25.0001, 137.9998) -> (-28.4202, 128.6029)
  line L46 (24.9999, 137.9998) -> (28.4202, 128.6029)
  line L47 (15.4, 137.9999) -> (8.4, 137.9999) construction
  line L48 (24.9999, 137.9998) -> (5.0007, 137.9998) construction
  line L49 (-0.0001, 137.9998) -> (24.9999, 137.9998)
  line L50 (24.9999, 137.9998) -> (-4.9989, 137.9998) construction
  line L51 (-0.0001, 137.9998) -> (-25.0001, 137.9998)
  line L52 (-0.0001, 137.9998) -> (-25.0001, 137.9998) construction
  line L53 (-0.0001, 137.9998) -> (-25.0001, 137.9998) construction
  circle A17 centre (-15.3999, 130.9999) radius 1.6
  circle A18 centre (15.4, 130.9999) radius 1.6
  line L54 (-132.0115, 47.3492) -> (-125.5836, 39.6889)
  line L55 (-107.0115, 90.6505) -> (-97.1634, 88.914)
  line L56 (-111.8115, 82.3367) -> (-115.3115, 76.2745) construction
  line L57 (-107.0115, 90.6505) -> (-117.0111, 73.3307) construction
  line L58 (-119.5115, 68.9999) -> (-107.0115, 90.6505)
  line L59 (-107.0115, 90.6505) -> (-122.0109, 64.6707) construction
  line L60 (-119.5115, 68.9999) -> (-132.0115, 47.3492)
  line L61 (-119.5115, 68.9999) -> (-132.0115, 47.3492) construction
  line L62 (-119.5115, 68.9999) -> (-132.0115, 47.3492) construction
  circle A19 centre (-121.1493, 52.1632) radius 1.6
  circle A20 centre (-105.7493, 78.8367) radius 1.6
  line L63 (-107.0114, -90.6507) -> (-97.1634, -88.9142)
  line L64 (-132.0114, -47.3494) -> (-125.5836, -39.689)
  line L65 (-127.2115, -55.6633) -> (-123.7115, -61.7255) construction
  line L66 (-132.0114, -47.3494) -> (-122.0118, -64.6693) construction
  line L67 (-119.5114, -69.0001) -> (-132.0114, -47.3494)
  line L68 (-132.0114, -47.3494) -> (-117.012, -73.3292) construction
  line L69 (-119.5114, -69.0001) -> (-107.0114, -90.6507)
  line L70 (-119.5114, -69.0001) -> (-107.0114, -90.6507) construction
  line L71 (-119.5114, -69.0001) -> (-107.0114, -90.6507) construction
  circle A21 centre (-105.7494, -78.8368) radius 1.6
  circle A22 centre (-121.1493, -52.1632) radius 1.6
  line L72 (-28.4202, -128.6031) -> (-97.1634, -88.9142)
  line L73 (97.1633, -88.9142) -> (28.4201, -128.6031)
  line L74 (125.5835, 39.6888) -> (125.5835, -39.689)
  line L75 (28.4202, 128.6029) -> (97.1634, 88.914)
  line L76 (-97.1634, 88.914) -> (-28.4202, 128.6029)
  line L77 (-125.5836, -39.689) -> (-125.5836, 39.6889)
  line L78 (-15.4, -131) -> (42.1, -131) construction
  circle A23 centre (15.4, -73.5001) radius 1.65
  circle A24 centre (-15.4001, -73.5) radius 1.65
  circle A25 centre (71.3528, -23.4133) radius 1.65
  circle A26 centre (55.9528, -50.0869) radius 1.65
  circle A27 centre (55.9528, 50.0867) radius 1.65
  circle A28 centre (71.3528, 23.413) radius 1.65
  circle A29 centre (-15.4, 73.4999) radius 1.65
  circle A30 centre (15.4, 73.4999) radius 1.65
  circle A31 centre (-71.3529, 23.4131) radius 1.65
  circle A32 centre (-55.9528, 50.0867) radius 1.65
  circle A33 centre (-55.9529, -50.0869) radius 1.65
  circle A34 centre (-71.3529, -23.4132) radius 1.65
  line L79 (30, -0.0001) -> (30, -10.9001)
  line L80 (30, -0.0001) -> (40.9, -0.0001) construction
  line L81 (-30, -0.0001) -> (-30, -10.9001)
  line L82 (30, -10.9001) -> (23.62, -21.9505)
  line L83 (30, -10.9001) -> (42.76, -10.9001) construction
  line L84 (23.62, -21.9505) -> (23.62, -30.6505)
  line L85 (23.62, -21.9505) -> (32.32, -21.9505) construction
  line L86 (23.62, -30.6505) -> (16.8489, -38.72)
  line L87 (23.62, -30.6505) -> (34.154, -30.6505) construction
  line L88 (16.8489, -38.72) -> (6.3489, -38.72)
  line L89 (6.3489, -38.72) -> (4.4205, -36.4219)
  line L90 (4.4205, -36.4219) -> (0, -36.4219)
  line L91 (-4.4205, -36.4219) -> (0, -36.4219)
  line L92 (-6.3489, -38.7201) -> (-4.4205, -36.4219)
  line L93 (-16.8489, -38.7201) -> (-6.3489, -38.7201)
  line L94 (-23.62, -30.6506) -> (-16.8489, -38.7201)
  line L95 (-23.62, -21.9506) -> (-23.62, -30.6506)
  line L96 (-30, -10.9001) -> (-23.62, -21.9506)
  line L97 (-30, -0.0001) -> (-30, -10.9001)
  line L98 (30, -0.0001) -> (30, 10.8999)
  line L99 (30, 10.8999) -> (23.62, 21.9504)
  line L100 (23.62, 21.9504) -> (23.62, 30.6504)
  line L101 (23.62, 30.6504) -> (16.8488, 38.7199)
  line L102 (16.8488, 38.7199) -> (6.3488, 38.7199)
  line L103 (6.3488, 38.7199) -> (4.4205, 36.4218)
  line L104 (4.4205, 36.4218) -> (0, 36.4218)
  line L105 (-16.8489, 38.7199) -> (-6.3489, 38.7199)
  line L106 (-6.3489, 38.7199) -> (-4.4205, 36.4218)
  line L107 (-4.4205, 36.4218) -> (0, 36.4218)
  line L108 (-23.62, 30.6504) -> (-16.8489, 38.7199)
  line L109 (-23.62, 21.9504) -> (-23.62, 30.6504)
  line L110 (-30, 10.8999) -> (-23.62, 21.9504)
  line L111 (-30, -0.0001) -> (-30, 10.8999)
  line L112 (-30, -0.0001) -> (-30, 10.8999)
  line L113 (0, -88.9499) -> (6, -88.9499)
  line L114 (6, -88.9499) -> (8.5, -88.9499) construction
  line L115 (6, -88.9499) -> (7.9151, -90.5569)
  line L116 (6, -88.9499) -> (8.5, -88.9499) construction
  line L117 (7.9151, -90.5569) -> (14.9151, -90.5569)
  line L118 (14.9151, -90.5569) -> (24.9151, -107.8774)
  line L119 (14.9151, -90.5569) -> (34.9151, -90.5569) construction
  line L120 (24.9151, -107.8774) -> (19.1301, -114.7719)
  line L121 (24.9151, -115.3493) -> (33.9151, -115.3493) construction
  line L122 (19.1301, -114.7719) -> (13.35, -114.7719)
  line L123 (19.1301, -114.7719) -> (24.9101, -114.7719) construction
  line L124 (13.35, -114.7719) -> (11.1, -110.8748)
  line L125 (13.35, -114.7719) -> (17.85, -114.7719) construction
  line L126 (11.1, -110.8748) -> (0, -110.8748)
  line L127 (-11.1, -110.8748) -> (0, -110.8748)
  line L128 (-13.35, -114.7719) -> (-17.85, -114.7719) construction
  line L129 (-19.13, -114.7719) -> (-13.35, -114.7719)
  line L130 (0, -88.9499) -> (-6, -88.95)
  line L131 (-6, -88.95) -> (-7.9151, -90.557)
  line L132 (-6, -88.95) -> (-8.5, -88.95) construction
  line L133 (-6, -88.95) -> (-8.5, -88.95) construction
  line L134 (-7.9151, -90.557) -> (-14.9151, -90.557)
  line L135 (-19.13, -114.7719) -> (-24.91, -114.7719) construction
  line L136 (-24.9151, -107.8775) -> (-19.13, -114.7719)
  line L137 (-14.9151, -90.557) -> (-24.9151, -107.8775)
  line L138 (-14.9151, -90.557) -> (-34.9151, -90.557) construction
  line L139 (-13.35, -114.7719) -> (-11.1, -110.8748)
  line L140 (101.5703, -45.8245) -> (96.0203, -55.4374)
  line L141 (90.4703, -65.0503) -> (96.0203, -55.4374)
  line L142 (92.7203, -68.9474) -> (90.4703, -65.0503)
  line L143 (92.7203, -68.9474) -> (90.4703, -72.8445) construction
  line L144 (70.967, -58.1954) -> (60.967, -75.5159) construction
  line L145 (89.8303, -73.953) -> (86.9403, -78.9587) construction
  line L146 (80.967, -75.5159) -> (89.8303, -73.953)
  line L147 (89.8303, -73.953) -> (92.7203, -68.9474)
  line L148 (70.967, -58.1954) -> (80.967, -75.5159)
  line L149 (77.0328, -44.475) -> (74.0329, -49.6712)
  line L150 (74.0329, -49.6712) -> (72.7829, -51.8362) construction
  line L151 (74.0329, -49.6712) -> (72.7829, -51.8362) construction
  line L152 (74.0329, -49.6712) -> (74.467, -52.1332)
  line L153 (74.467, -52.1332) -> (70.967, -58.1954)
  line L154 (108.9603, -40.8188) -> (111.8503, -35.8132) construction
  line L155 (105.882, -32.3616) -> (108.9603, -40.8188)
  line L156 (85.882, -32.3616) -> (95.882, -15.0411) construction
  line L157 (85.882, -32.3616) -> (105.882, -32.3616)
  line L158 (108.9603, -40.8188) -> (106.0703, -45.8245)
  line L159 (106.0703, -45.8245) -> (108.3203, -41.9274) construction
  line L160 (106.0703, -45.8245) -> (101.5703, -45.8245)
  line L161 (80.0328, -39.2789) -> (81.2828, -37.1138) construction
  line L162 (80.0328, -39.2789) -> (82.382, -38.4238)
  line L163 (80.0328, -39.2789) -> (81.2828, -37.1138) construction
  line L164 (77.0328, -44.475) -> (80.0328, -39.2789)
  line L165 (82.382, -38.4238) -> (85.882, -32.3616)
  line L166 (90.4702, 65.0502) -> (96.0202, 55.4373)
  line L167 (101.5702, 45.8244) -> (96.0202, 55.4373)
  line L168 (106.0702, 45.8244) -> (101.5702, 45.8244)
  line L169 (106.0702, 45.8244) -> (108.3202, 41.9273) construction
  line L170 (85.8821, 32.3615) -> (95.8821, 15.041) construction
  line L171 (108.9603, 40.8188) -> (111.8503, 35.8131) construction
  line L172 (105.8821, 32.3615) -> (108.9603, 40.8188)
  line L173 (108.9603, 40.8188) -> (106.0702, 45.8244)
  line L174 (85.8821, 32.3615) -> (105.8821, 32.3615)
  line L175 (77.0328, 44.4748) -> (80.0328, 39.2788)
  line L176 (80.0328, 39.2788) -> (81.2828, 37.1137) construction
  line L177 (80.0328, 39.2788) -> (81.2828, 37.1137) construction
  line L178 (80.0328, 39.2788) -> (82.3821, 38.4237)
  line L179 (82.3821, 38.4237) -> (85.8821, 32.3615)
  line L180 (89.8302, 73.953) -> (86.9402, 78.9586) construction
  line L181 (80.9669, 75.5157) -> (89.8302, 73.953)
  line L182 (70.9669, 58.1952) -> (60.9669, 75.5157) construction
  line L183 (70.9669, 58.1952) -> (80.9669, 75.5157)
  line L184 (89.8302, 73.953) -> (92.7202, 68.9473)
  line L185 (92.7202, 68.9473) -> (90.4702, 72.8444) construction
  line L186 (92.7202, 68.9473) -> (90.4702, 65.0502)
  line L187 (74.0328, 49.671) -> (72.7828, 51.8361) construction
  line L188 (74.0328, 49.671) -> (74.4669, 52.133)
  line L189 (74.0328, 49.671) -> (72.7828, 51.8361) construction
  line L190 (77.0328, 44.4748) -> (74.0328, 49.671)
  line L191 (74.4669, 52.133) -> (70.9669, 58.1952)
  line L192 (-11.1001, 110.8746) -> (-0.0001, 110.8746)
  line L193 (11.0999, 110.8746) -> (-0.0001, 110.8746)
  line L194 (13.3499, 114.7717) -> (11.0999, 110.8746)
  line L195 (13.3499, 114.7717) -> (17.8499, 114.7717) construction
  line L196 (14.915, 90.5568) -> (34.915, 90.5568) construction
  line L197 (19.13, 114.7717) -> (24.91, 114.7717) construction
  line L198 (24.915, 107.8773) -> (19.13, 114.7717)
  line L199 (19.13, 114.7717) -> (13.3499, 114.7717)
  line L200 (14.915, 90.5568) -> (24.915, 107.8773)
  line L201 (0, 88.9498) -> (5.9999, 88.9498)
  line L202 (5.9999, 88.9498) -> (8.4999, 88.9498) construction
  line L203 (5.9999, 88.9498) -> (8.4999, 88.9498) construction
  line L204 (5.9999, 88.9498) -> (7.915, 90.5568)
  line L205 (7.915, 90.5568) -> (14.915, 90.5568)
  line L206 (-19.1301, 114.7717) -> (-24.9102, 114.7717) construction
  line L207 (-24.9151, 107.8773) -> (-19.1301, 114.7717)
  line L208 (-14.9151, 90.5567) -> (-34.9151, 90.5567) construction
  line L209 (-14.9151, 90.5567) -> (-24.9151, 107.8773)
  line L210 (-19.1301, 114.7717) -> (-13.3501, 114.7717)
  line L211 (-13.3501, 114.7717) -> (-17.8501, 114.7717) construction
  line L212 (-13.3501, 114.7717) -> (-11.1001, 110.8746)
  line L213 (-6, 88.9498) -> (-8.5001, 88.9498) construction
  line L214 (-6, 88.9498) -> (-7.9151, 90.5567)
  line L215 (-6, 88.9498) -> (-8.5, 88.9498) construction
  line L216 (0, 88.9498) -> (-6, 88.9498)
  line L217 (-7.9151, 90.5567) -> (-14.9151, 90.5567)
  line L218 (-101.5703, 45.8243) -> (-96.0203, 55.4372)
  line L219 (-90.4703, 65.0501) -> (-96.0203, 55.4372)
  line L220 (-92.7203, 68.9472) -> (-90.4703, 65.0501)
  line L221 (-92.7203, 68.9472) -> (-90.4703, 72.8443) construction
  line L222 (-70.9671, 58.1952) -> (-60.9671, 75.5157) construction
  line L223 (-89.8303, 73.9529) -> (-86.9403, 78.9585) construction
  line L224 (-80.9671, 75.5157) -> (-89.8303, 73.9529)
  line L225 (-89.8303, 73.9529) -> (-92.7203, 68.9472)
  line L226 (-70.9671, 58.1952) -> (-80.9671, 75.5157)
  line L227 (-77.0329, 44.4748) -> (-74.0329, 49.671)
  line L228 (-74.0329, 49.671) -> (-72.7829, 51.8361) construction
  line L229 (-74.0329, 49.671) -> (-72.7829, 51.8361) construction
  line L230 (-74.0329, 49.671) -> (-74.4671, 52.133)
  line L231 (-74.4671, 52.133) -> (-70.9671, 58.1952)
  line L232 (-108.9604, 40.8187) -> (-111.8504, 35.813) construction
  line L233 (-105.8821, 32.3615) -> (-108.9604, 40.8187)
  line L234 (-85.8821, 32.3615) -> (-95.8821, 15.041) construction
  line L235 (-85.8821, 32.3615) -> (-105.8821, 32.3615)
  line L236 (-108.9604, 40.8187) -> (-106.0703, 45.8243)
  line L237 (-106.0703, 45.8243) -> (-108.3203, 41.9272) construction
  line L238 (-106.0703, 45.8243) -> (-101.5703, 45.8243)
  line L239 (-80.0329, 39.2787) -> (-81.2829, 37.1136) construction
  line L240 (-80.0329, 39.2787) -> (-82.3821, 38.4236)
  line L241 (-80.0329, 39.2787) -> (-81.2829, 37.1136) construction
  line L242 (-77.0329, 44.4748) -> (-80.0329, 39.2787)
  line L243 (-82.3821, 38.4236) -> (-85.8821, 32.3615)
  line L244 (-90.4703, -65.0503) -> (-96.0203, -55.4375)
  line L245 (-101.5703, -45.8246) -> (-96.0203, -55.4375)
  line L246 (-106.0703, -45.8246) -> (-101.5703, -45.8246)
  line L247 (-106.0703, -45.8246) -> (-108.3203, -41.9275) construction
  line L248 (-85.8821, -32.3617) -> (-95.8821, -15.0412) construction
  line L249 (-108.9603, -40.8189) -> (-111.8503, -35.8133) construction
  line L250 (-105.8821, -32.3617) -> (-108.9603, -40.8189)
  line L251 (-108.9603, -40.8189) -> (-106.0703, -45.8246)
  line L252 (-85.8821, -32.3617) -> (-105.8821, -32.3617)
  line L253 (-77.0329, -44.475) -> (-80.0329, -39.2789)
  line L254 (-80.0329, -39.2789) -> (-81.2829, -37.1139) construction
  line L255 (-80.0329, -39.2789) -> (-81.2829, -37.1139) construction
  line L256 (-80.0329, -39.2789) -> (-82.3821, -38.4239)
  line L257 (-82.3821, -38.4239) -> (-85.8821, -32.3617)
  line L258 (-89.8303, -73.9531) -> (-86.9402, -78.9588) construction
  line L259 (-80.967, -75.5159) -> (-89.8303, -73.9531)
  line L260 (-70.967, -58.1954) -> (-60.967, -75.5159) construction
  line L261 (-70.967, -58.1954) -> (-80.967, -75.5159)
  line L262 (-89.8303, -73.9531) -> (-92.7203, -68.9475)
  line L263 (-92.7203, -68.9475) -> (-90.4703, -72.8446) construction
  line L264 (-92.7203, -68.9475) -> (-90.4703, -65.0503)
  line L265 (-74.0329, -49.6712) -> (-72.7829, -51.8363) construction
  line L266 (-74.0329, -49.6712) -> (-74.467, -52.1332)
  line L267 (-74.0329, -49.6712) -> (-72.7829, -51.8362) construction
  line L268 (-77.0329, -44.475) -> (-74.0329, -49.6712)
  line L269 (-74.467, -52.1332) -> (-70.967, -58.1954)
  line L270 (0, -88.9499) -> (0, -36.4219)
  line L271 (0, -91.9499) -> (5.9999, -91.9499)
  line L272 (5.9999, -91.9499) -> (7.532, -93.2355)
  line L273 (5.9999, -91.9499) -> (7.9999, -91.9499) construction
  line L274 (7.532, -93.2355) -> (12.532, -93.2355)
  line L275 (12.532, -93.2355) -> (20.032, -106.2259)
  line L276 (20.032, -106.2259) -> (16.8181, -110.0561)
  line L277 (16.8181, -110.0561) -> (13.8181, -110.0561)
  line L278 (13.8181, -110.0561) -> (12.5681, -107.8911)
  line L279 (12.5681, -107.8911) -> (0, -107.8911)
  line L280 (-6, -91.9499) -> (-8, -91.9499) construction
  line L281 (0, -91.9499) -> (-6, -91.9499)
  line L282 (-7.5321, -93.2355) -> (-12.5321, -93.2355)
  line L283 (-6, -91.9499) -> (-7.5321, -93.2355)
  line L284 (-12.5321, -93.2355) -> (-20.0321, -106.2259)
  line L285 (-13.8181, -110.0561) -> (-12.5681, -107.8911)
  line L286 (-16.8181, -110.0561) -> (-13.8181, -110.0561)
  line L287 (-20.0321, -106.2259) -> (-16.8181, -110.0561)
  line L288 (-12.5681, -107.8911) -> (0, -107.8911)
  line L289 (79.6309, -45.975) -> (76.6309, -51.1711)
  line L290 (76.9782, -53.1407) -> (74.4782, -57.4709)